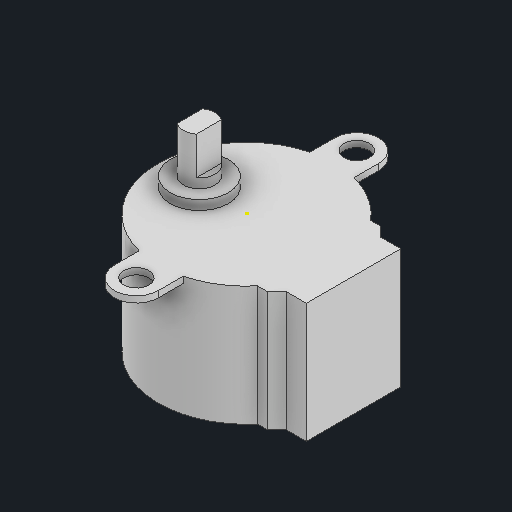
# Autodesk Inventor part: stepper_motor
Saved by Autodesk Inventor 2026.2 (Build 302298000, 298)
## iProperties
Created: 2025-12-19
Part Number: stepper_motor
Material: Generic
Document SubType Name: Modeling
Designer: colin
Density: 1 g/cm^3
Appearance: Default
Author: colin
Autodesk Inventor part; units mm, degrees
ref_plane "YZ Plane" through (0, 0, 0) normal (1, 0, 0) x (0, 1, 0)
ref_plane "XZ Plane" through (0, 0, 0) normal (0, 1, 0) x (-1, 0, 0)
ref_plane "XY Plane" through (0, 0, 0) normal (0, 0, 1) x (1, 0, 0)
sketch "Sketch1" plane through (0, 0, 0) normal (0, 1, 0) x (-1, 0, 0)
  line L0 (-12.2941, 0) -> (-17, 0)
  line L1 (-17, 0) -> (-17, 7.5)
  line L2 (0, 0) -> (-12.2941, 0)
  line L3 (-12.2941, 9) -> (-10.7238, 9)
  line L4 (-12.2941, 9) -> (-13.7941, 7.5)
  line L5 (-12.2941, 9) -> (-9.8817, 9) construction
  arc A0 (-10.7238, -9) -> (-10.7238, 9) centre (0, 0) ccw
  line L6 (-17, 7.5) -> (-13.7941, 7.5)
  line L7 (-17, 0) -> (-17, -7.5)
  line L8 (-12.2941, -9) -> (-10.7238, -9)
  line L9 (-12.2941, -9) -> (-13.7941, -7.5)
  line L10 (-12.2941, -9) -> (-9.8817, -9) construction
  line L11 (-17, -7.5) -> (-13.7941, -7.5)
  dimension "d3" = 9
  dimension "d4" = 135
  constraints: 24 end point, 5 symmetric about line, 3 horizontal, 2 parallel, 2 point on circle, 2 point on line, 1 centre point, 1 coincident, 1 perpendicular
  measures "d3" distance of L0.start L3.start
  measures "d4" angle of L4 L5
extrude "Extrusion1" add sketch "Sketch1" along normal blind 19
sketch "Sketch2" plane through (0, 19, 0) normal (0, 1, 0) x (1, 0, 0)
  circle A0 centre (-7.5, 0) radius 4.6
  circle A1 centre (-7.5, 0) radius 2.5
  arc A2 (10.7238, 9) -> (10.7238, -9) centre (0, 0) ccw projected
  line L0 (-6, -2) -> (-6, 2)
  line L1 (-9, 2) -> (-9, -2)
  circle A3 centre (0, -17.5) radius 2
  arc A4 (-3.5, -17.5) -> (3.5, -17.5) centre (0, -17.5) ccw
  line L2 (-3.5, -17.5) -> (-3.5, -13.5554)
  line L3 (3.5, -17.5) -> (3.5, -13.5554)
  arc A5 (-3.5, -13.5554) -> (3.5, -13.5554) centre (0, 0) ccw
  line L4 (0, 0) -> (2, 0)
  arc A6 (10.7238, 9) -> (10.7238, -9) centre (0, 0) ccw
  circle A7 centre (0, 17.5) radius 2
  arc A8 (3.5, 17.5) -> (-3.5, 17.5) centre (0, 17.5) ccw
  line L5 (-3.5, 17.5) -> (-3.5, 13.5554)
  line L6 (3.5, 17.5) -> (3.5, 13.5554)
  arc A9 (3.5, 13.5554) -> (-3.5, 13.5554) centre (0, 0) ccw
  point P0 (-7.5, -3.3735)
  dimension "d7" = 5
  dimension "d8" = 9.2
  dimension "d9" = 0
  dimension "d10" = 7.5
  dimension "d12" = 0
  dimension "d13" = 3
  dimension "d14" = 4
  dimension "d15" = 0
  dimension "d16" = 17.5
  dimension "d17" = 7
  constraints: 18 point on circle, 14 end point, 9 centre point, 8 symmetric about line, 2 coincident, 2 concentric, 2 parallel, 2 tangent, 1 horizontal, 1 vertical, 4 other
  measures "d7" diameter of A1
  measures "d8" diameter of A0
  measures "d9" vertical distance of point (0, 0) A0.centre
  measures "d10" distance of A2.centre A0.centre
  measures "d12" horizontal distance of A0.centre point (-7.5, -3.374)
  measures "d13" distance between parallel lines of L1 L0
  measures "d14" diameter of A3
  measures "d15" horizontal distance of point (0, 0) A3.centre
  measures "d16" distance of point (0, 0) A3.centre
  measures "d17" diameter of A4
extrude "Extrusion2" add sketch "Sketch2" against normal blind 1 contours A2 L3 A4 L2 | A2 L5 A8 L6
extrude "Extrusion3" add sketch "Sketch2" along normal blind 9 contours L0 A1 L1
extrude "Extrusion4" add sketch "Sketch2" along normal blind 3 contours A1 L0 | L0 A1 L1 | L1 A1
extrude "Extrusion5" add sketch "Sketch2" along normal blind 1.5 contours A0
sketch "Sketch4" plane through (0, 19, 0) normal (0, 1, 0) x (1, 0, 0)
  point P0 (0, 0)
body "Solid1"
